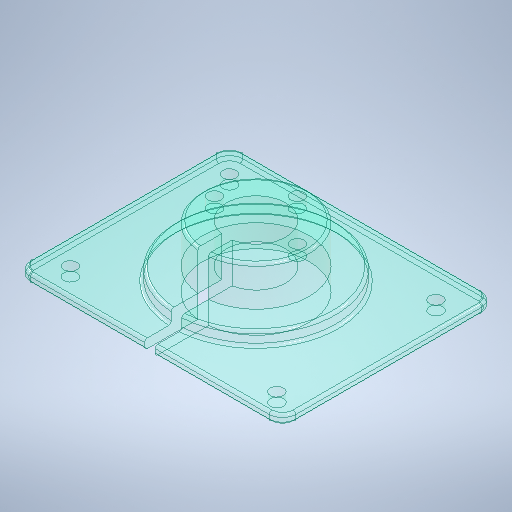
# Autodesk Inventor part: Table_Filter
Saved by Autodesk Inventor 2025.2 (Build 292293000, 293)
## iProperties
Created: 2025-05-24
Part Number: Table_Filter
Material: PBT Plastic
Document SubType Name: Modeling
Designer: Musa Gamal
Density: 1.31 g/cm^3
Appearance: Indoor Pool
Author: Musa Gamal
Autodesk Inventor part; units mm, degrees
ref_plane "YZ Plane" through (0, 0, 0) normal (1, 0, 0) x (0, 1, 0)
ref_plane "XZ Plane" through (0, 0, 0) normal (0, 1, 0) x (-1, 0, 0)
ref_plane "XY Plane" through (0, 0, 0) normal (0, 0, 1) x (1, 0, 0)
sketch "Sketch1" plane through (0, 0, 0) normal (0, 1, 0) x (-1, 0, 0)
  arc A0 (-3.8355, -211.5136) -> (4.1645, -211.5136) centre (0.1645, -251.3131) ccw
  arc A1 (-3.8355, -211.5136) -> (4.1645, -211.5136) centre (0.1645, -251.3131) ccw
  line L0 (4.1645, -211.5136) -> (4.1645, -196.0639)
  line L1 (4.1645, -171.3131) -> (4.1645, -211.5136)
  line L2 (-3.8355, -211.5136) -> (-3.8355, -197.7163)
  line L3 (4.1645, -171.3131) -> (90.1645, -171.3131)
  line L4 (100.1645, -181.3131) -> (100.1645, -321.3131)
  line L5 (90.1645, -331.3131) -> (-89.8355, -331.3131)
  line L6 (-99.8355, -321.3131) -> (-99.8355, -181.3131)
  line L7 (-89.8355, -171.3131) -> (0.1645, -171.3131)
  circle A2 centre (80.1645, -311.3131) radius 5
  circle A3 centre (80.1645, -191.3131) radius 5
  circle A4 centre (-79.8355, -187.0663) radius 5
  circle A5 centre (-79.8355, -307.0663) radius 5
  line L8 (-3.8355, -211.5136) -> (-3.8355, -171.3131)
  arc A6 (90.1645, -331.3131) -> (100.1645, -321.3131) centre (90.1645, -321.3131) ccw
  arc A7 (100.1645, -181.3131) -> (90.1645, -171.3131) centre (90.1645, -181.3131) ccw
  arc A8 (-89.8355, -171.3131) -> (-99.8355, -181.3131) centre (-89.8355, -181.3131) ccw
  arc A9 (-99.8355, -321.3131) -> (-89.8355, -331.3131) centre (-89.8355, -321.3131) ccw
  point P0 (0, 0)
  point P1 (-43.9118, -267.1712)
  point P2 (100.1645, -171.3131)
  point P3 (100.1645, -331.3131)
  point P4 (-99.8355, -331.3131)
  point P5 (-99.8355, -171.3131)
  dimension "d0" = 80
  dimension "d1" = 160
  dimension "d2" = 200
  dimension "d3" = 10
  dimension "d4" = 10
  dimension "d5" = 10
  dimension "d6" = 10
  dimension "d7" = 20
  dimension "d8" = 120
  dimension "d9" = 160
  dimension "d10" = 20
  dimension "d11" = 120
  dimension "d12" = 160
  dimension "d13" = 100
  dimension "d14" = 10
  constraints: 18 end point, 12 point on circle, 10 centre point, 10 point on line, 8 tangent, 4 equal radius, 3 perpendicular, 2 horizontal, 1 coincident, 1 vertical
  measures "d0" distance of A1.centre L7.end
  measures "d1" distance of point (100.165, -171.313) point (100.165, -331.313)
  measures "d2" distance of point (100.165, -331.313) point (-99.835, -331.313)
  measures "d3" diameter of A2
  measures "d4" diameter of A3
  measures "d5" diameter of A4
  measures "d6" diameter of A5
  measures "d7" distance from line of A2.centre L5
  measures "d8" distance of A2.centre A3.centre
  measures "d9" horizontal distance of A5.centre A2.centre
  measures "d10" distance from line of A2.centre L4
  measures "d11" distance of A5.centre A4.centre
  measures "d12" horizontal distance of A3.centre A4.centre
  measures "d13" distance from line of L6 A0.centre
  measures "d14" radius of A6
extrude "Extrusion1" add sketch "Sketch1" along normal blind 7
sketch "Sketch2" plane through (0, 7, 0) normal (0, 1, 0) x (1, 0, 0)
  line L0 (99.8355, 181.3131) -> (99.8355, 321.3131) projected
  arc A0 (99.8355, 321.3131) -> (89.8355, 331.3131) centre (89.8355, 321.3131) ccw projected
  line L1 (89.8355, 331.3131) -> (-90.1645, 331.3131) projected
  arc A1 (-90.1645, 331.3131) -> (-100.1645, 321.3131) centre (-90.1645, 321.3131) ccw projected
  line L2 (-100.1645, 321.3131) -> (-100.1645, 181.3131) projected
  arc A2 (-100.1645, 181.3131) -> (-90.1645, 171.3131) centre (-90.1645, 181.3131) ccw projected
  line L3 (-90.1645, 171.3131) -> (-4.1645, 171.3131) projected
  line L4 (-4.1645, 171.3131) -> (-4.1645, 211.5136) projected
  arc A3 (3.8355, 211.5136) -> (-4.1645, 211.5136) centre (-0.1645, 251.3131) ccw projected
  line L5 (3.8355, 211.5136) -> (3.8355, 171.3131) projected
  line L6 (3.8355, 171.3131) -> (89.8355, 171.3131) projected
  arc A4 (89.8355, 171.3131) -> (99.8355, 181.3131) centre (89.8355, 181.3131) ccw projected
  circle A5 centre (-80.1645, 191.3131) radius 5 projected
  circle A6 centre (-80.1645, 311.3131) radius 5 projected
  circle A7 centre (79.8355, 307.0663) radius 5 projected
  circle A8 centre (79.8355, 187.0663) radius 5 projected
  arc A9 (3.8355, 191.4466) -> (-4.1645, 191.4466) centre (-0.1645, 251.3131) ccw
  point P0 (0, 0)
  dimension "d17" = 120
  constraints: 2 point on circle, 2 point on line, 1 centre point, 1 coincident
  measures "d17" diameter of A9
extrude "Extrusion2" add sketch "Sketch2" along normal blind 10 contours L5 A3 L4 A9
sketch "Sketch3" plane through (0, 17, 0) normal (0, 1, 0) x (1, 0, 0)
  line L0 (3.8355, 211.5136) -> (3.8355, 191.4466) projected
  arc A0 (3.8355, 191.4466) -> (-4.1645, 191.4466) centre (-0.1645, 251.3131) ccw projected
  line L1 (-4.1645, 191.4466) -> (-4.1645, 211.5136) projected
  arc A1 (3.8355, 211.5136) -> (-4.1645, 211.5136) centre (-0.1645, 251.3131) ccw projected
  arc A2 (3.8355, 211.5136) -> (-4.1645, 211.5136) centre (-0.1645, 251.3131) ccw
  circle A3 centre (-0.1645, 251.3131) radius 40
  point P0 (0, 0)
  constraints: 2 centre point, 2 end point, 2 point on circle, 1 coincident, 1 concentric
extrude "Extrusion3" add sketch "Sketch3" along normal blind 30 contours A3 A1
sketch "Sketch4" plane through (-0.1645, 47, -251.3131) normal (0, 1, 0) x (1, 0, 0)
  circle A0 centre (0, 0) radius 40 projected
  circle A1 centre (0, 0) radius 27.5
  circle A2 centre (0, 0) radius 22.4
  line L0 (4, -39.7995) -> (4, -59.8665) projected
  arc A3 (4, -59.8665) -> (-4, -59.8665) centre (0, 0) ccw projected
  line L1 (-4, -59.8665) -> (-4, -39.7995) projected
  arc A4 (4, -39.7995) -> (-4, -39.7995) centre (0, 0) ccw projected
  line L2 (-4, -59.8665) -> (-4, 0)
  line L3 (-4, 0) -> (0, 0)
  line L4 (0, 0) -> (4, 0)
  line L5 (4, -59.8665) -> (4, 0)
  point P0 (0.1645, -251.3131)
  point P1 (4, -22.04)
  point P2 (-4, -22.04)
  dimension "d23" = 55
  dimension "d24" = 44.8
  dimension "d27" = 4
  constraints: 8 end point, 3 point on line, 2 centre point, 2 coincident, 2 perpendicular
  measures "d23" diameter of A1
  measures "d24" diameter of A2
  measures "d27" distance of L2.end L3.end
extrude "Extrusion4" cut sketch "Sketch4" against normal through all contours L2 L3 L4 L5 A2 | A2 L5 L4 L3 L2
extrude "Extrusion5" cut sketch "Sketch4" against normal through all contours L2 A1 L5 A0 | L2 A2 L5 A1 picked at (3.1125, -31.4915) picked at (-3.1132, -23.8691)
sketch "Sketch5" plane through (0, 47, 0) normal (0, 1, 0) x (1, 0, 0)
  line L0 (-4.1645, 211.5136) -> (-4.1645, 229.2731) projected
  arc A0 (3.8355, 229.2731) -> (-4.1645, 229.2731) centre (-0.1645, 251.3131) ccw projected
  line L1 (3.8355, 229.2731) -> (3.8355, 211.5136) projected
  arc A1 (3.8355, 211.5136) -> (-4.1645, 211.5136) centre (-0.1645, 251.3131) ccw projected
  line L2 (-0.1645, 251.3131) -> (-0.1645, 282.5131)
  circle A2 centre (-0.1645, 282.5131) radius 5
  circle A3 centre (31.0355, 251.3131) radius 5
  circle A4 centre (-31.3645, 251.3131) radius 5
  point P0 (0, 0)
  dimension "d33" = 31.2
  dimension "d34" = 10
  dimension "d35" = 10
  dimension "d36" = 10
  dimension "d37" = 31.2
  dimension "d38" = 31.2
  constraints: 3 centre point, 2 end point, 1 coincident, 1 vertical
  measures "d33" distance of L2.start L2.end
  measures "d34" diameter of A2
  measures "d35" diameter of A3
  measures "d36" diameter of A4
  measures "d37" distance of A0.centre A3.centre
  measures "d38" distance of A0.centre A4.centre
extrude "Extrusion6" cut sketch "Sketch5" against normal blind 8 contours A2 | A3 | A4
fillet "Fillet1" radius 2 2 edges at (-0.1645, 7, -311.3131) (-0.1645, 17, -311.3131)
fillet "Fillet2" radius 2 19 edges at (-0.1645, 47, -291.3131) (-0.1645, 7, -331.3131) (-97.2356, 7, -328.3841) (-100.1645, 7, -251.3131) (-97.2356, 7, -174.242) (-47.1645, 7, -171.3131) (99.8355, 7, -251.3131) (96.9065, 7, -174.242) (46.8355, 7, -171.3131) (96.9065, 7, -328.3841) (99.8355, 0, -251.3131) (96.9065, 0, -328.3841) (-0.1645, 0, -331.3131) (-97.2356, 0, -328.3841) (-100.1645, 0, -251.3131) (-97.2356, 0, -174.242) (-47.1645, 0, -171.3131) (46.8355, 0, -171.3131) (96.9065, 0, -174.242)
equation "\"d13\" = 0.5 * d2"
equation "\"d37\" = d33"
equation "\"d38\" = d33"
body "Solid1"
